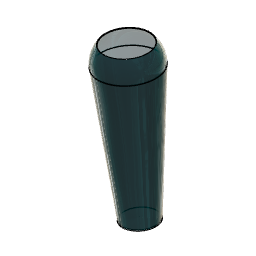
bottle v1 (Autodesk Fusion 360 design; units mm, degrees)
Autodesk Fusion 360 part; units mm, degrees
sketch "Sketch1" plane through (0, 0, 0) normal (0, 1, 0) x (1, 0, 0)
  line L0 (0, 0) -> (50.2955, 0)
  line L1 (50.2955, -399.7131) -> (50.2955, 0)
  arc A0 (25.1478, -455.6829) -> (50.2955, -399.7131) centre (-24.5625, -399.7131) ccw
  arc A1 (23.8196, -454.1875) -> (48.2955, -399.7131) centre (-24.5625, -399.7131) ccw
  line L2 (48.2955, -399.7131) -> (48.2955, -2)
  line L3 (0, -2) -> (48.2955, -2)
  line L4 (25.1478, -455.6829) -> (23.8196, -454.1875)
  line L5 (-54.645, -596.0155) -> (0, 0) construction
  line L6 (0, 0) -> (0, -2)
  dimension "d1" = 2
  constraint coincident L0.start L5.end
  constraint horizontal L0
  constraint perpendicular L0 L1
  constraint tangent L1 A0
  constraint perpendicular L3 L6
revolve "Revolve1" add sketch "Sketch1" angle 360 about axis through (-54.645, 0, 596.0155) along (0.091301, 0, -0.995823)
